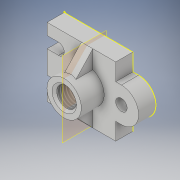
# Autodesk Inventor part: основ4ание
Saved by Autodesk Inventor 2019.4 (Build 234330000, 330)
## iProperties
Created: 2020-04-20
Part Number: основ4ание
Material: Типовые
Document SubType Name: Modeling
Designer: Asus
Density: 1 g/cm^3
Appearance: По умолчанию
Mass: 63.2584 g
Surface Area: 165.139 cm^2
Volume: 63.2584 cm^3
Author: Asus
Autodesk Inventor part; units mm, degrees
ref_plane "XZ Plane" through (0, 0, 0) normal (0, 1, 0) x (-1, 0, 0)
sketch "Эскиз1" plane through (0, 0, 0) normal (0, 0, 1) x (1, 0, 0)
  line L0 (60, -60) -> (0, -60)
  line L1 (0, -10) -> (0, 0)
  line L2 (60, -60) -> (0, -60)
  line L3 (60, 0) -> (60, -15)
  arc A0 (65, -45) -> (65, -15) centre (65, -30) ccw
  line L4 (60, 0) -> (60, -15)
  line L5 (60, -45) -> (60, -60)
  line L6 (65, -15) -> (60, -15)
  line L7 (65, -45) -> (60, -45)
  circle A1 centre (65, -30) radius 5
  line L8 (0, -60) -> (0, -50)
  line L9 (0, -60) -> (0, -50)
  line L10 (0, -40) -> (0, -20)
  line L11 (0, -40) -> (0, -20)
  line L12 (0, -10) -> (0, 0)
  line L13 (0, -10) -> (10, -10)
  line L14 (10, -20) -> (0, -20)
  line L15 (0, 0) -> (60, 0)
  line L16 (0, 0) -> (15, 0)
  arc A2 (10, -20) -> (10, -10) centre (10, -15) ccw
  line L17 (0, -50) -> (10, -50)
  line L18 (10, -40) -> (0, -40)
  arc A3 (10, -50) -> (10, -40) centre (10, -45) ccw
  constraints: 38 end point, 7 parallel, 6 point on circle, 4 centre point, 3 horizontal, 1 coincident, 1 perpendicular, 1 point on line
extrude "Выдавливание1" add sketch "Эскиз1" along normal blind 15
sketch "Эскиз3" plane through (0, 0, 15) normal (0, 0, 1) x (1, 0, 0)
  line L0 (60, 0) -> (0, 0) projected
  circle A0 centre (34.8659, -30) radius 15
  constraints: 1 centre point, 1 coincident
extrude "Выдавливание2" add sketch "Эскиз3" along normal blind 20
sketch "Эскиз4" plane through (0, 0, 0) normal (0, 0, 1) x (1, 0, 0)
  circle A0 centre (34.8659, -30) radius 15
  circle A1 centre (34.8659, -30) radius 15 projected
  circle A2 centre (65, -30) radius 5 projected
  line L0 (0, 0) -> (0, -10) projected
  line L1 (0, -10) -> (10, -10) projected
  arc A3 (10, -20) -> (10, -10) centre (10, -15) ccw projected
  line L2 (10, -20) -> (0, -20) projected
  line L3 (0, -20) -> (0, -40) projected
  line L4 (0, -40) -> (10, -40) projected
  arc A4 (10, -50) -> (10, -40) centre (10, -45) ccw projected
  line L5 (10, -50) -> (0, -50) projected
  line L6 (0, -50) -> (0, -60) projected
  line L7 (0, -60) -> (60, -60) projected
  line L8 (60, -60) -> (60, -45) projected
  line L9 (60, -45) -> (65, -45) projected
  arc A5 (65, -45) -> (65, -15) centre (65, -30) ccw projected
  line L10 (65, -15) -> (60, -15) projected
  line L11 (60, -15) -> (60, 0) projected
  line L12 (60, 0) -> (0, 0) projected
  constraints: 1 centre point
ref_plane "РабПлоскость1" through (0, 0, 35) normal (0, 0, 1) x (1, 0, 0)
sketch "Эскиз6" plane through (0, 0, 35) normal (0, 0, 1) x (1, 0, 0)
  point P0 (60, 0)
  point P1 (35, -30)
  point P2 (35, -30)
  point P3 (35, -30)
  constraints: 2 coincident
hole "Отверстие1" at (35, -30, 35) direction (0, 0, -1) diameter 17.3 depth 35 tip angle 118
chamfer "Фаска1" distance 2 angle 45 1 edges at (35, -21.35, 35)
sketch "Эскиз7" plane through (0, 0, 0) normal (0, 1, 0) x (-1, 0, 0)
  point P0 (0, 0)
ref_plane "РабПлоскость2" through (35, 0, 0) normal (1, 0, 0) x (0, 1, 0)
sketch "Эскиз10" plane through (35, 0, 0) normal (1, 0, 0) x (0, 1, 0)
  line L0 (-16.0535, 30) -> (0, 15)
  line L1 (-16.0535, 30) -> (-16.0535, 15)
  line L2 (-15, 15) -> (-15, 35) projected
  point P0 (0, 0)
  point P1 (-60, 15)
  dimension "d37" = 15
  dimension "d52" = 15
  constraints: 4 end point, 1 coincident
  measures "d37" horizontal distance of point (-15, 35) point (0, 15)
  measures "d52" distance of L0.start L1.end
extrude "Ребро жесткости1" add sketch "Эскиз10" along normal mid plane 10 rib yes fills toward (-8.0609, 22.4635) open curves L0 L1
sketch "Эскиз12" plane through (35, 0, 0) normal (1, 0, 0) x (0, 1, 0)
  line L0 (-44.2259, 30) -> (-60, 15)
  line L1 (-44.2259, 30) -> (-44.2259, 15)
  line L2 (-15, 35) -> (-45, 35) projected
  point P0 (0, 0)
  dimension "d51" = 5
  constraints: 4 end point, 1 coincident, 1 vertical
  measures "d51" distance from line of L0.start L2
extrude "Ребро жесткости2" add sketch "Эскиз12" along normal mid plane 10 rib yes fills toward (-44.2759, 22.5) open curves L1 L0
